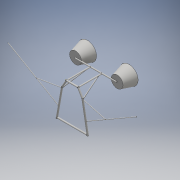
# Autodesk Inventor part: Part4
Saved by Autodesk Inventor 2016 (Build 200138000, 138)
## iProperties
Created: 2016-05-15
Part Number: Part4
Material: Generic
Document SubType Name: Modeling
Designer: Mauricio
Density: 1 g/cm^3
Appearance: Default
Author: Mauricio
Autodesk Inventor part; units mm, degrees
sketch "Sketch1" plane through (0, 0, 0) normal (1, 0, 0) x (0, 1, 0)
  circle A0 centre (0, 0) radius 25
  dimension "d0" = 50
  constraints: 1 centre point, 1 coincident
  measures "d0" diameter of A0
extrude "Extrusion1" add sketch "Sketch1" along normal blind 420
sketch "Sketch2" plane through (0, 0, 0) normal (0, 1, 0) x (-1, 0, 0)
  point P0 (0, 0)
sketch "Sketch3" plane through (0, 0, 0) normal (0, 1, 0) x (-1, 0, 0)
  line L0 (-400.246418, 0) -> (-426.916088, 15.397741)
  line L1 (-400.246418, 0) -> (-369.450936, 0) construction
  point P0 (0, 0)
  dimension "d3" = 150
  constraints: 4 end point, 1 equal length, 1 horizontal
  measures "d3" angle of L1 L0
sketch "Sketch4" plane through (420, 0, 0) normal (1, 0, 0) x (0, 0, -1)
  circle A0 centre (0, 0) radius 25 projected
  line L0 (0, -25) -> (0, 25)
  constraints: 2 end point, 2 point on circle, 1 vertical
ref_plane "Work Plane1" through (400.246418, 0, 0) normal (-0.5, 0, 0.8660254) x (0.8660254, 0, 0.5)
sketch "Sketch6" plane through (0, 0, 0) normal (0, 1, 0) x (-1, 0, 0)
  line L0 (0, 0) -> (32.070817, 18.516095)
  line L1 (0, 0) -> (37.032189, 0) construction
  dimension "d5" = 30
  constraints: 4 end point, 1 equal length, 1 horizontal
  measures "d5" angle of L1 L0
ref_plane "Work Plane2" through (0, 0, 0) normal (-0.5, 0, -0.8660254) x (-0.8660254, 0, 0.5)
sketch "Sketch7" plane through (400.246418, 0, 0) normal (-0.5, 0, 0.8660254) x (0.8660254, 0, 0.5)
  ellipse E0 centre (17.107104, 0) end of major axis (17.107104, -25) minor radius 12.5
  line L0 (29.607104, 0) -> (-20.392896, 0)
  circle A0 centre (4.607104, 0) radius 25
  point P0 (-346.623566, 0)
  dimension "d23" = 50
  constraints: 2 end point, 2 horizontal alignment, 1 horizontal, 1 midpoint, 3 other
  measures "d23" distance of L0.start L0.end
sketch "Sketch8" plane through (0, 0, 0) normal (-0.5, 0, -0.8660254) x (-0.8660254, 0, 0.5)
  ellipse E0 centre (0, 0) end of major axis (0, -25) minor radius 12.5 projected
  line L0 (12.5, 0) -> (-12.5, 0)
  circle A0 centre (-12.5, 0) radius 25
  dimension "d15" = 25
  constraints: 2 end point, 1 coincident, 1 horizontal alignment, 5 other
  measures "d15" distance of L0.start L0.end
extrude "Extrusion3" add sketch "Sketch8" along normal blind 300 and the other way blind 20 contours A0 E0 L0 | L0 E0 A0 | A0 E0 picked at (-19.633519, -6.766459)
extrude "Extrusion4" add sketch "Sketch7" against normal blind 300 and the other way blind 11 contours A0 E0 L0 | L0 E0 A0 | A0 L0 E0 | E0 L0 A0
sketch "Sketch10" plane through (0, 0, 0) normal (0, 1, 0) x (-1, 0, 0)
  line L0 (-575.886922, -245.004069) -> (-532.585652, -270.004069)
  line L1 (-532.585652, -270.004069) -> (-557.476245, -265.615186)
  line L2 (-532.585652, -270.004069) -> (-507.311081, -270.004069) construction
  point P0 (0, 0)
  dimension "d29" = 170
  constraints: 4 end point, 1 equal length, 1 horizontal
  measures "d29" angle of L2 L1
ref_plane "Work Plane6" through (532.585652, 0, -270.004069) normal (-0.1736482, 0, 0.9848078) x (0.9848078, 0, 0.1736482)
sketch "Sketch11" plane through (0, 0, 0) normal (0, 1, 0) x (-1, 0, 0)
  line L0 (117.763855, -278.469011) -> (137.46001, -274.996047)
  line L1 (117.763855, -278.469011) -> (137.763855, -278.469011) construction
  point P0 (0, 0)
  dimension "d31" = 20
  dimension "d32" = 10
  constraints: 4 end point, 1 equal length, 1 horizontal
  measures "d31" distance of L0.start L0.end
  measures "d32" angle of L1 L0
ref_plane "Work Plane7" through (-117.763855, 0, -278.469011) normal (-0.1736482, 0, -0.9848078) x (-0.9848078, 0, 0.1736482)
sketch "Sketch13" plane through (532.585652, 0, -270.004069) normal (-0.1736482, 0, 0.9848078) x (0.9848078, 0, 0.1736482)
  ellipse E0 centre (23.492316, 0) end of major axis (23.492316, 25) minor radius 23.492316
  line L0 (46.984631, 0) -> (21.984631, 0)
  circle A0 centre (21.984631, 0) radius 25
  point P0 (-477.608765, 0)
  dimension "d35" = 25
  constraints: 2 end point, 2 horizontal alignment, 1 coincident, 1 horizontal, 3 other
  measures "d35" distance of L0.start L0.end
extrude "Extrusion5" add sketch "Sketch13" along normal blind 18 and the other way blind 1000 contours A0 E0 | E0 A0 | A0 E0 picked at (15.784017, 0.835556) picked at (31.582888, -23.082688) picked at (-0.819464, 1.859813)
sketch "Sketch14" plane through (-117.763855, 0, -278.469011) normal (-0.1736482, 0, -0.9848078) x (-0.9848078, 0, 0.1736482)
  ellipse E0 centre (23.240764, 0) end of major axis (23.240764, -25) minor radius 23.492316
  line L0 (46.73308, 0) -> (21.73308, 0)
  circle A0 centre (21.73308, 0) radius 25
  point P0 (-67.619121, 0)
  dimension "d41" = 25
  constraints: 2 end point, 2 horizontal alignment, 1 coincident, 1 horizontal, 3 other
  measures "d41" distance of L0.start L0.end
extrude "Extrusion6" add sketch "Sketch14" along normal blind 1000 and the other way blind 18 contours A0 E0 | A0 E0 picked at (15.532466, 0.835556) picked at (-1.071015, 1.859814)
sketch "Sketch15" plane through (0, 0, 0) normal (0, 1, 0) x (-1, 0, 0)
  point P0 (0, 0)
sketch "Sketch16" plane through (0, 0, 0) normal (1, 0, 0) x (0, 1, 0)
  line L0 (0, -1256.171103) -> (0, -1231.171103)
  circle A0 centre (0, -1231.171103) radius 25
  point P0 (0, 0)
  dimension "d46" = 25
  constraints: 2 end point, 1 coincident, 1 vertical, 1 vertical alignment, 2 other
  measures "d46" distance of L0.start L0.end
extrude "Extrusion7" add sketch "Sketch16" along normal blind 708.75 and the other way blind 306.375
ref_plane "Work Plane8" through (752.504658, 0, -1246.653027) normal (0.9848078, 0, 0.1736482) x (0, 1, 0)
sketch "Sketch17" plane through (752.504658, 0, -1246.653027) normal (0.9848078, 0, 0.1736482) x (0, 1, 0)
  line L0 (-25, 0) -> (25, 0) projected
  line L1 (0, 0) -> (0, 400)
  circle A0 centre (0, 400) radius 10
  point P0 (0, 1358.384629)
  point P1 (7.038536, 0)
  point P2 (-7.038536, 0)
  dimension "d51" = 400
  dimension "d52" = 20
  constraints: 2 end point, 1 centre point, 1 coincident, 1 midpoint, 1 vertical
  measures "d51" distance of L1.start L1.end
  measures "d52" diameter of A0
sketch "Sketch18" plane through (0, 0, 0) normal (0, 1, 0) x (-1, 0, 0)
  point P0 (0, 0)
sketch "Sketch19" plane through (0, 0, 0) normal (0, 1, 0) x (-1, 0, 0)
  line L0 (-683.035487, -852.612562) -> (-546.53698, -616.190212)
  line L1 (-683.035487, -852.612562) -> (-410.038472, -852.612562) construction
  point P0 (0, 0)
  dimension "d53" = 60
  constraints: 4 end point, 1 equal length, 1 horizontal
  measures "d53" angle of L1 L0
ref_plane "Work Plane9" through (683.035487, 0, -852.612562) normal (-0.8660254, 0, -0.5) x (-0.5, 0, 0.8660254)
sketch "Sketch20" plane through (683.035487, 0, -852.612562) normal (-0.8660254, 0, -0.5) x (-0.5, 0, 0.8660254)
  circle A0 centre (0, 0) radius 10
  point P0 (1079.901881, 0)
  dimension "d55" = 20
  constraints: 1 centre point
  measures "d55" diameter of A0
extrude "Extrusion8" add sketch "Sketch20" against normal blind 1950 and the other way blind 5
sketch "Sketch21" plane through (0, 0, 0) normal (0, 1, 0) x (-1, 0, 0)
  line L0 (338.004192, -1253.70191) -> (267.743534, -859.920956)
  line L1 (160.825318, -253.557621) -> (337.435132, -1255.16165)
  line L2 (267.743534, -859.920956) -> (55.112629, -491.633427)
  line L3 (267.743534, -859.920956) -> (693.005342, -859.920956) construction
  point P0 (0, 0)
  dimension "d60" = 400
  dimension "d61" = 120
  constraints: 6 end point, 1 equal length, 1 horizontal, 1 point on line
  measures "d60" distance of L0.start L0.end
  measures "d61" angle of L3 L2
ref_plane "Work Plane10" through (-267.743534, 0, -859.920956) normal (-0.8660254, 0, 0.5) x (0.5, 0, 0.8660254)
sketch "Sketch22" plane through (-267.743534, 0, -859.920956) normal (-0.8660254, 0, 0.5) x (0.5, 0, 0.8660254)
  circle A0 centre (0, 0) radius 10
  point P0 (878.58516, 0)
  dimension "d63" = 20
  constraints: 1 centre point
  measures "d63" diameter of A0
extrude "Extrusion9" add sketch "Sketch22" along normal blind 1950
sketch "Sketch23" plane through (0, 0, 0) normal (0, 1, 0) x (-1, 0, 0)
  line L0 (-752.504658, -1246.653027) -> (-575.886922, -245.004069)
  line L1 (-681.166011, -842.071453) -> (-582.186602, -280.731332)
  line L2 (-582.186602, -280.731332) -> (-607.804417, -184.068373)
  line L3 (265.895608, -849.440851) -> (1951.493071, 123.739298)
  line L4 (265.895608, -849.440851) -> (166.916147, -288.100432)
  line L5 (160.825318, -253.557621) -> (337.435132, -1255.16165)
  line L6 (166.916147, -288.100432) -> (191.587493, -148.182273)
  point P0 (0, 0)
  dimension "d66" = 100
  dimension "d71" = 570
  constraints: 8 end point, 4 point on line
  measures "d66" distance of L1.end L2.end
  measures "d71" distance of L4.start L4.end
ref_plane "Work Plane11" through (582.186602, 0, -280.731332) normal (-0.9666296, 0, 0.2561781) x (0.2561781, 0, 0.9666296)
sketch "Sketch24" plane through (582.186602, 0, -280.731332) normal (-0.9666296, 0, 0.2561781) x (0.2561781, 0, 0.9666296)
  circle A0 centre (0, 0) radius 10
  point P0 (122.21973, 0)
  dimension "d68" = 20
  constraints: 1 centre point
  measures "d68" diameter of A0
extrude "Extrusion10" add sketch "Sketch24" against normal blind 774.25
ref_plane "Work Plane12" through (-166.916147, 0, -288.100432) normal (-0.9848078, 0, -0.1736482) x (-0.1736482, 0, 0.9848078)
sketch "Sketch25" plane through (-166.916147, 0, -288.100432) normal (-0.9848078, 0, -0.1736482) x (-0.1736482, 0, 0.9848078)
  circle A0 centre (0, 0) radius 10
  point P0 (254.738854, 0)
  dimension "d73" = 20
  constraints: 1 centre point
  measures "d73" diameter of A0
extrude "Extrusion11" add sketch "Sketch25" along normal blind 846.5 and the other way blind 30.75
sketch "Sketch26" plane through (0, 0, 0) normal (0, 1, 0) x (-1, 0, 0)
  line L0 (-391.132487, -25) -> (-405.566243, 0)
  circle A0 centre (-405.566243, 0) radius 20
  point P0 (0, 0)
  dimension "d78" = 40
  constraints: 1 centre point
  measures "d78" diameter of A0
extrude "Extrusion12" add sketch "Sketch26" along normal blind 800
sketch "Sketch27" plane through (0, 0, 0) normal (0, 1, 0) x (-1, 0, 0)
  circle A0 centre (-15.392671, 0) radius 20
  point P0 (0, 0)
  dimension "d82" = 40
  constraints: 1 centre point
  measures "d82" diameter of A0
extrude "Extrusion13" add sketch "Sketch27" along normal blind 800
sketch "Sketch28" plane through (0, 0, 0) normal (1, 0, 0) x (0, 1, 0)
  line L0 (800, -20) -> (800, 20) projected
  circle A0 centre (800, 0) radius 20
  point P0 (0, 0)
  constraints: 1 midpoint, 1 vertical alignment, 2 other
extrude "Extrusion14" add sketch "Sketch28" along normal blind 900 and the other way blind 500
sketch "Sketch29" plane through (0, 0, 0) normal (0, 0, 1) x (1, 0, 0)
  circle A0 centre (406.461405, 684.020717) radius 15
  point P0 (0, 0)
  dimension "d89" = 30
  constraints: 1 centre point
  measures "d89" diameter of A0
sketch "Sketch30" plane through (0, 0, 0) normal (0, 1, 0) x (-1, 0, 0)
  circle A0 centre (-558.501414, -277.620326) radius 15
  point P0 (0, 0)
  dimension "d90" = 30
  constraints: 1 centre point
  measures "d90" diameter of A0
loft "Loft1" add profiles "Sketch30", "Sketch29"
sketch "Sketch31" plane through (0, 0, 0) normal (0, 0, 1) x (1, 0, 0)
  circle A0 centre (14.263983, 707.832615) radius 15
  point P0 (0, 0)
  dimension "d95" = 30
  constraints: 1 centre point
  measures "d95" diameter of A0
sketch "Sketch32" plane through (0, 0, 0) normal (0, 1, 0) x (-1, 0, 0)
  circle A0 centre (142.793601, -292.413549) radius 15
  point P0 (0, 0)
  dimension "d96" = 30
  constraints: 1 centre point
  measures "d96" diameter of A0
loft "Loft2" add profiles "Sketch32", "Sketch31"
ref_plane "Work Plane13" through (0, 815, 0) normal (0, 1, 0) x (-1, 0, 0)
sketch "Sketch33" plane through (0, 815, 0) normal (0, 1, 0) x (-1, 0, 0)
  line L0 (-900, 20) -> (-900, -20) projected
  circle A0 centre (-900, 0) radius 200
  point P0 (0, 0)
  dimension "d102" = 400
  constraints: 1 centre point, 1 midpoint
  measures "d102" diameter of A0
extrude "Extrusion15" add sketch "Sketch33" along normal blind 400 draft 15
sketch "Sketch35" plane through (0, 815, 0) normal (0, 1, 0) x (-1, 0, 0)
  line L0 (500, -20) -> (500, 20) projected
  circle A0 centre (500, 0) radius 200
  point P0 (0, 0)
  dimension "d112" = 400
  constraints: 1 centre point, 1 midpoint
  measures "d112" diameter of A0
extrude "Extrusion16" add sketch "Sketch35" along normal blind 400 draft 15
sketch "Sketch37" plane through (0, 0, 0) normal (1, 0, 0) x (0, 1, 0)
  point P0 (0, 0)
sketch "Sketch38" plane through (900, 1215, 0) normal (0, 1, 0) x (1, 0, 0)
  circle A0 centre (0, 0) radius 300
  point P0 (-900, 0)
  dimension "d122" = 600
  constraints: 1 centre point
  measures "d122" diameter of A0
extrude "Extrusion17" cut sketch "Sketch38" against normal blind 380 draft -15
sketch "Sketch39" plane through (-500, 1215, 0) normal (0, 1, 0) x (1, 0, 0)
  circle A0 centre (0, 0) radius 300
  point P0 (500, 0)
  dimension "d125" = 600
  constraints: 1 centre point
  measures "d125" diameter of A0
extrude "Extrusion18" cut sketch "Sketch39" against normal blind 380 draft -15
sketch "Sketch40" plane through (0, 0, 0) normal (0, 0, 1) x (1, 0, 0)
  point P0 (0, 0)
body "Solid1"
